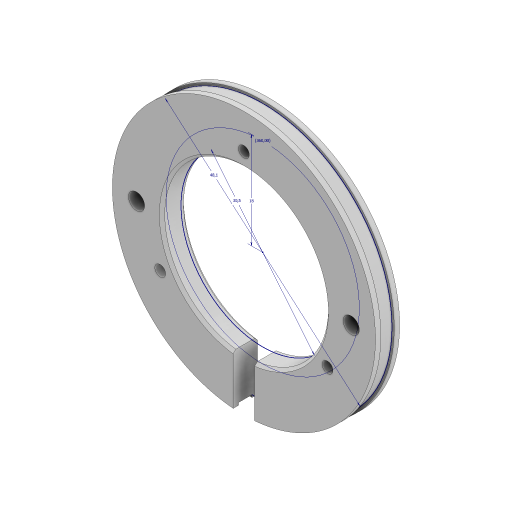
# Autodesk Inventor part: Adapter-MitutoyoMT1-SM2-v3(flex)
Saved by Autodesk Inventor 2023 (Build 270158000, 158)
## iProperties
Created: 2023-09-27
Part Number: Adapter-MitutoyoMT1-SM2-v3(flex)
Material: Generic
Document SubType Name: Modeling
Designer: spim-user
Density: 1 g/cm^3
Appearance: Default
Author: spim-user
Autodesk Inventor part; units mm, degrees
ref_plane "YZ Plane" through (0, 0, 0) normal (1, 0, 0) x (0, 1, 0)
ref_plane "XZ Plane" through (0, 0, 0) normal (0, 1, 0) x (-1, 0, 0)
ref_plane "XY Plane" through (0, 0, 0) normal (0, 0, 1) x (1, 0, 0)
sketch "Sketch1" plane through (0, 0, 0) normal (0, 0, 1) x (1, 0, 0)
  circle A0 centre (0, 0) radius 15.25
  circle A1 centre (0, 0) radius 24.05
  point P0 (0, 18)
  point P1 (-15.5885, -9)
  point P2 (15.5885, -9)
  dimension "d0" = 30.5
  dimension "d1" = 48.1
  dimension "d2" = 18
  dimension "d5" = 360
  constraints: 2 centre point, 2 coincident, 4 other
  measures "d0" diameter of A0
  measures "d1" diameter of A1
  measures "d2" distance of point (0, 0) point (0, 18)
extrude "Extrusion1" add sketch "Sketch1" along normal blind 2.5
hole "Hole1" at (0, 18, 0) at (-15.5885, -9, 0) at (15.5885, -9, 0) direction (0, 0, 1) diameter 2 end through all
sketch "Sketch2" plane through (0, 0, 2.5) normal (0, 0, 1) x (1, 0, 0)
  circle A0 centre (0, 0) radius 24.5
  circle A1 centre (0, 18) radius 1 projected
  circle A2 centre (0, 0) radius 15.25 projected
  circle A3 centre (-15.5885, -9) radius 1 projected
  circle A4 centre (15.5885, -9) radius 1 projected
  dimension "d16" = 49
  constraints: 1 centre point, 1 coincident
  measures "d16" diameter of A0
extrude "Extrusion2" add sketch "Sketch2" along normal blind 1
sketch "Sketch3" plane through (0, 0, 0) normal (0, 0, -1) x (-1, 0, 0)
  circle A0 centre (0, 0) radius 24.5
  circle A1 centre (0, 18) radius 1 projected
  circle A2 centre (0, 0) radius 15.25 projected
  circle A3 centre (-15.5885, -9) radius 1 projected
  circle A4 centre (15.5885, -9) radius 1 projected
  dimension "d21" = 49
  constraints: 1 centre point, 1 coincident
  measures "d21" diameter of A0
extrude "Extrusion3" add sketch "Sketch3" along normal blind 1
sketch "Sketch4" plane through (0, 0, 3.5) normal (0, 0, 1) x (1, 0, 0)
  line L0 (2, -30.8109) -> (-2, -30.8109)
  line L1 (-2, -30.8109) -> (-2, -10.8109)
  line L2 (-2, -10.8109) -> (2, -10.8109)
  line L3 (2, -10.8109) -> (2, -30.8109)
  line L4 (2, -30.8109) -> (-2, -10.8109) construction
  line L5 (-2, -30.8109) -> (2, -10.8109) construction
  line L6 (0, -41.8731) -> (0, 35.5622) projected
  point P0 (0, 0)
  point P1 (0, -20.8109)
  dimension "d22" = 4
  dimension "d23" = 20
  dimension "d33" = 0
  constraints: 12 end point, 2 midpoint, 2 parallel, 1 horizontal, 1 perpendicular
  measures "d22" distance of L1.end L2.end
  measures "d23" distance of L0.end L1.end
  measures "d33" distance from line of L6 point (0, -20.811)
extrude "Extrusion4" cut sketch "Sketch4" against normal through all
sketch "Sketch5" plane through (0, 0, 3.5) normal (0, 0, 1) x (1, 0, 0)
  point P0 (0, 0)
  point P1 (-20, 0)
  point P2 (20, 0)
hole "Hole2" at (-20, 0, 3.5) at (20, 0, 3.5) direction (0, 0, -1) diameter 3 end through all
chamfer "Chamfer1" distance 0.5 angle 45 2 edges at (0, 15.25, 3.5) (0, 15.25, -1)
body "Solid1"
